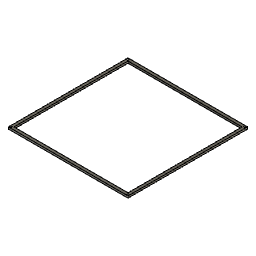
Front of Frame v5 (Autodesk Fusion 360 design; units mm, degrees)
Autodesk Fusion 360 part; units mm, degrees
sketch "Sketch1" plane through (0, 0, 0) normal (0, 0, 1) x (1, 0, 0)
  line L0 (-80, 75) -> (140, 75)
  line L1 (140, 75) -> (140, -145)
  line L2 (140, -145) -> (-80, -145)
  line L3 (-80, -145) -> (-80, 75)
  line L4 (-75, 70) -> (135, 70)
  line L5 (135, 70) -> (135, -140)
  line L6 (135, -140) -> (-75, -140)
  line L7 (-75, -140) -> (-75, 70)
  circle A0 centre (137.5, 72.5) radius 1.5
  circle A1 centre (137.5, -142.5) radius 1.5
  circle A2 centre (-77.5, -142.5) radius 1.5
  circle A3 centre (-77.5, 72.5) radius 1.5
  dimension "d1" = 220
  dimension "d2" = 220
  dimension "d3" = 5
  dimension "d4" = 5
  dimension "d5" = 5
  dimension "d6" = 5
  dimension "d7" = 3
  dimension "d8" = 3
  dimension "d9" = 3
  dimension "d10" = 3
  dimension "d11" = 2.5
  dimension "d12" = 2.5
  dimension "d13" = 2.5
  dimension "d14" = 2.5
  dimension "d15" = 2.5
  dimension "d16" = 2.5
  dimension "d17" = 2.5
  dimension "d18" = 2.5
  dimension "d19" = 210
  dimension "d20" = 210
  constraint horizontal L0
  constraint vertical L1
  constraint horizontal L2
  constraint vertical L3
  constraint horizontal L4
  constraint vertical L5
  constraint horizontal L6
  constraint vertical L7
  measures "d1" distance of L0.start L0.end
  measures "d2" distance of L0.start L2.end
  measures "d3" distance of L3 L7
  measures "d4" distance of L1 L5
  measures "d5" distance of L0 L4
  measures "d6" distance of L2 L6
  measures "d7" diameter of A0
  measures "d8" diameter of A1
  measures "d9" diameter of A2
  measures "d10" diameter of A3
  measures "d11" distance of L0 A3.centre
  measures "d12" distance of L3 A3.centre
  measures "d13" distance of L1 A0.centre
  measures "d14" distance of L0 A0.centre
  measures "d15" distance of L1 A1.centre
  measures "d16" distance of L2 A1.centre
  measures "d17" distance of L3 A2.centre
  measures "d18" distance of L2 A2.centre
  measures "d19" distance of L4.end L5.end
  measures "d20" distance of L4.start L4.end
extrude "Extrude1" add sketch "Sketch1" along normal blind 3.5
